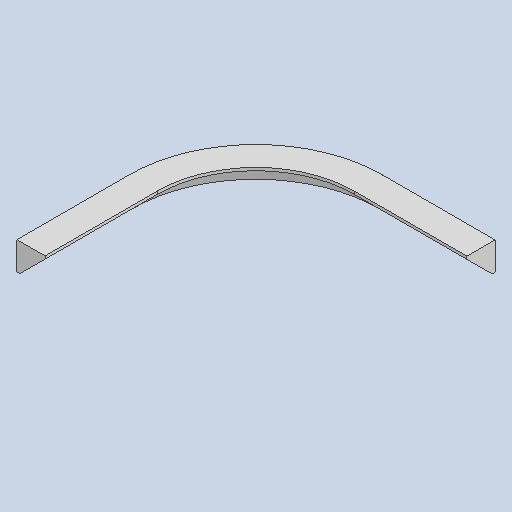
# Autodesk Inventor part: test1
Saved by Autodesk Inventor 2025 (Build 290162000, 162)
## iProperties
Created: 2025-04-20
Part Number: test1
Material: Generic
Document SubType Name: Sheet Metal
Designer: Pravoslav
Density: 1 g/cm^3
Sheet Metal Rule: Default_mm
Appearance: Default
Author: Pravoslav
Autodesk Inventor part; units mm, degrees
ref_plane "YZ Plane" through (0, 0, 0) normal (1, 0, 0) x (0, 1, 0)
ref_plane "XZ Plane" through (0, 0, 0) normal (0, 1, 0) x (-1, 0, 0)
ref_plane "XY Plane" through (0, 0, 0) normal (0, 0, 1) x (1, 0, 0)
sketch "Sketch1" plane through (0, 0, 0) normal (0, 1, 0) x (-1, 0, 0)
  circle A0 centre (0, 0) radius 45
  circle A1 centre (0, 0) radius 35
  line L0 (35, 0) -> (45, 0)
  line L1 (45, 0) -> (45, 40)
  line L2 (45, 40) -> (35, 40)
  line L3 (35, 40) -> (35, 0)
  line L4 (-0.1589, -34.9996) -> (-40.1589, -34.9996)
  line L5 (-40.1589, -34.9996) -> (-40.1589, -44.9997)
  line L6 (-40.1589, -44.9997) -> (-0.1589, -44.9997)
  line L7 (-0.1589, -44.9997) -> (-0.1589, -34.9996)
  point P0 (-0.1589, -44.9997)
  point P1 (45, 0)
  point P2 (-28.2847, -34.9996)
  point P3 (35, 28.2843)
  point P4 (-0.1589, -44.9997)
  dimension "d0" = 90
  dimension "d1" = 70
  dimension "d2" = 40
  dimension "d3" = 40
  constraints: 16 end point, 4 parallel, 4 point on circle, 2 centre point, 2 coincident, 2 horizontal, 2 perpendicular
  measures "d0" diameter of A0
  measures "d1" diameter of A1
  measures "d2" distance of L1.end L0.end
  measures "d3" distance of L6.end L5.end
extrude "Extrusion1" add sketch "Sketch1" along normal blind 10 contours L7 A1 L0 A0 | L6 L5 L4 A0 | A0 L4 L7 | L0 L3 A0 | A0 L3 L2 L1
chamfer "Chamfer1" distance 9 angle 45 3 edges at (-35, 0, 20) (-24.6925, 0, -24.8048) (20.1589, 0, -34.9996)
equation "\"BendRadius\" = Thickness"
equation "\"BendReliefWidth\" = Thickness"
equation "\"BendReliefDepth\" = 0.5 * Thickness"
equation "\"CornerReliefSize\" = 4 * Thickness"
equation "\"MinimumRemnant\" = 2 * Thickness"
equation "\"TransitionRadius\" = BendRadius"
equation "\"JacobiRadiusSize\" = BendRadius"
equation "\"GapSize\" = Thickness"
equation "\"Thickness\" = 0.5"
body "Solid1"
